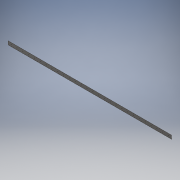
# Autodesk Inventor part: Long Hinge
Saved by Autodesk Inventor 2018 (Build 220112000, 112)
## iProperties
Created: 2018-10-30
Part Number: Long Hinge
Material: Steel
Document SubType Name: Modeling
Designer: P301319
Density: 7.85 g/cm^3
Appearance: Semi-Polished
Author: P301319
Autodesk Inventor part; units mm, degrees
ref_plane "YZ Plane" through (0, 0, 0) normal (1, 0, 0) x (0, 1, 0)
ref_plane "XZ Plane" through (0, 0, 0) normal (0, 1, 0) x (-1, 0, 0)
ref_plane "XY Plane" through (0, 0, 0) normal (0, 0, 1) x (1, 0, 0)
sketch "Sketch1" plane through (0, 0, 0) normal (1, 0, 0) x (0, 1, 0)
  line L0 (0, 0) -> (1, 0)
  line L1 (1, 0) -> (1, -30)
  line L2 (1, -30) -> (0, -30)
  line L3 (0, -30) -> (0, 0)
  circle A0 centre (2.5, -30) radius 1.25
  circle A1 centre (2.5, -30) radius 1.75
  dimension "d0" = 1
  dimension "d1" = 30
  dimension "d2" = 2.5
  dimension "d3" = 2.5
  dimension "d4" = 3.5
  constraints: 8 end point, 2 centre point, 2 parallel, 1 coincident, 1 horizontal, 1 perpendicular, 1 point on line
  measures "d0" distance of L1.end L2.end
  measures "d1" distance of L0.end L1.end
  measures "d2" diameter of A0
  measures "d3" distance of L2.end A0.centre
  measures "d4" diameter of A1
extrude "Extrusion1" add sketch "Sketch1" along normal blind 1400
sketch "Sketch2" plane through (0, 0, 0) normal (0, 0, 1) x (1, 0, 0)
  line L0 (0, 1) -> (25, 1)
  line L1 (25, 1) -> (25, 4.25)
  line L2 (25, 4.25) -> (0, 4.25)
  line L3 (0, 4.25) -> (0, 1)
  point P0 (0, 0)
  dimension "d7" = 25
  dimension "d8" = 3.25
  constraints: 8 end point, 2 parallel, 1 horizontal, 1 perpendicular
  measures "d7" distance of L2.end L1.end
  measures "d8" distance of L1.end L0.end
extrude "Extrusion2" cut sketch "Sketch2" against normal through all
pattern_linear "Rectangular Pattern1" count 28 spacing 50 along (1, 0, 0) of "Extrusion2"
sketch "Sketch3" plane through (0, 1, 0) normal (0, 1, 0) x (1, 0, 0)
  line L0 (0, 0) -> (0, 30.9014) projected
  line L1 (0, 0) -> (1400, 0) projected
  point P0 (25, 15.4507)
  point P1 (0, 15.4507)
  point P2 (75, 15.4507)
  point P3 (125, 15.4507)
  point P4 (175, 15.4507)
  point P5 (225, 15.4507)
  point P6 (275, 15.4507)
  point P7 (325, 15.4507)
  point P8 (375, 15.4507)
  point P9 (425, 15.4507)
  point P10 (475, 15.4507)
  point P11 (525, 15.4507)
  point P12 (575, 15.4507)
  point P13 (625, 15.4507)
  point P14 (675, 15.4507)
  point P15 (725, 15.4507)
  point P16 (775, 15.4507)
  point P17 (825, 15.4507)
  point P18 (875, 15.4507)
  point P19 (925, 15.4507)
  point P20 (975, 15.4507)
  point P21 (1025, 15.4507)
  point P22 (1075, 15.4507)
  point P23 (1125, 15.4507)
  point P24 (1175, 15.4507)
  point P25 (1225, 15.4507)
  point P26 (1275, 15.4507)
  point P27 (1325, 15.4507)
  point P28 (1375, 15.4507)
  dimension "d14" = 25
  dimension "d17" = 50
  constraints: 1 horizontal, 1 horizontal alignment, 1 midpoint, 27 other
  measures "d14" distance from line of L0 point (25, 15.451)
  measures "d17" distance of point (25, 15.451) point (75, 15.451)
hole "Hole1" at (25, 1, -15.4507) at (75, 1, -15.4507) at (125, 1, -15.4507) at (175, 1, -15.4507) at (225, 1, -15.4507) at (275, 1, -15.4507) at (325, 1, -15.4507) at (375, 1, -15.4507) at (425, 1, -15.4507) at (475, 1, -15.4507) at (525, 1, -15.4507) at (575, 1, -15.4507) at (625, 1, -15.4507) at (675, 1, -15.4507) at (725, 1, -15.4507) at (775, 1, -15.4507) at (825, 1, -15.4507) at (875, 1, -15.4507) at (925, 1, -15.4507) at (975, 1, -15.4507) at (1025, 1, -15.4507) at (1075, 1, -15.4507) at (1125, 1, -15.4507) at (1175, 1, -15.4507) at (1225, 1, -15.4507) at (1275, 1, -15.4507) at (1325, 1, -15.4507) at (1375, 1, -15.4507) direction (0, -1, 0) diameter 3 end through all countersink diameter 5 countersink angle 90
body "Solid1"
